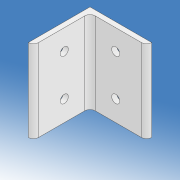
# Autodesk Inventor part: NASA-20-EBOX-EXT-CB-01
Saved by Autodesk Inventor 2020 (Build 240168000, 168)
## iProperties
Created: 2019-12-04
Part Number: NASA-20-EBOX-EXT-CB-01
Material: Generic
Document SubType Name: Modeling
Designer: mpark
Density: 1 g/cm^3
Appearance: White
Author: mpark
Autodesk Inventor part; units mm, degrees
ref_plane "YZ Plane" through (0, 0, 0) normal (1, 0, 0) x (0, 1, 0)
ref_plane "XZ Plane" through (0, 0, 0) normal (0, 1, 0) x (-1, 0, 0)
ref_plane "XY Plane" through (0, 0, 0) normal (0, 0, 1) x (1, 0, 0)
sketch "Sketch1" plane through (0, 0, 0) normal (0, 1, 0) x (-1, 0, 0)
  line L0 (-38.1, 0) -> (0, 0)
  line L1 (0, 0) -> (0, 38.1)
  line L2 (-34.925, 3.175) -> (-6.35, 3.175)
  line L3 (-3.175, 6.35) -> (-3.175, 34.925)
  line L4 (0, 38.1) -> (0, 38.1)
  line L5 (-38.1, 0) -> (-38.1, 0)
  arc A0 (0, 38.1) -> (-3.175, 34.925) centre (0, 34.925) ccw
  arc A1 (-34.925, 3.175) -> (-38.1, 0) centre (-34.925, 0) ccw
  arc A2 (-6.35, 3.175) -> (-3.175, 6.35) centre (-6.35, 6.35) ccw
  point P0 (0, 38.1)
  dimension "d0" = 38.1
  dimension "d1" = 38.1
  dimension "d2" = 3.175
  dimension "d3" = 3.175
  constraints: 12 end point, 6 point on circle, 6 tangent, 3 centre point, 3 perpendicular, 2 equal radius, 2 horizontal, 1 other
  measures "d0" distance of L0.end L1.end
  measures "d1" distance of L0.start L0.end
  measures "d2" distance between parallel lines of L0 L2
  measures "d3" radius of A0
extrude "Extrusion1" add sketch "Sketch1" along normal blind 50.8
sketch "Sketch2" plane through (38.1, 0, 0) normal (0, 0, -1) x (-1, 0, 0)
  line L0 (0, 0) -> (38.1, 0) projected
  line L1 (38.1, 0) -> (38.1, 50.8) projected
  line L2 (0, 50.8) -> (38.1, 50.8) projected
  line L3 (0, 0) -> (0, 50.8) projected
  point P0 (19.05, 38.1)
  point P1 (19.05, 12.7)
  dimension "d6" = 12.7
  dimension "d7" = 12.7
  dimension "d8" = 19.05
  constraints: 1 vertical alignment
  measures "d6" distance from line of point (19.05, 12.7) L0
  measures "d7" distance from line of L2 point (19.05, 38.1)
  measures "d8" distance from line of L1 point (19.05, 38.1)
hole "Hole1" at (19.05, 38.1, 0) at (19.05, 12.7, 0) direction (0, 0, 1) diameter 5 end through all
sketch "Sketch3" plane through (0, 0, 0) normal (-1, 0, 0) x (0, 0, 1)
  line L0 (0, 0) -> (38.1, 0) projected
  line L1 (38.1, 0) -> (38.1, 50.8) projected
  line L2 (0, 50.8) -> (38.1, 50.8) projected
  line L3 (0, 0) -> (0, 50.8) projected
  point P0 (19.05, 38.1)
  point P1 (19.05, 12.7)
  dimension "d16" = 12.7
  dimension "d17" = 12.7
  dimension "d18" = 19.05
  constraints: 1 vertical alignment
  measures "d16" distance from line of L2 point (19.05, 38.1)
  measures "d17" distance from line of L0 point (19.05, 12.7)
  measures "d18" distance from line of point (19.05, 38.1) L1
hole "Hole2" at (0, 38.1, 19.05) at (0, 12.7, 19.05) direction (1, 0, 0) diameter 5 end through all
equation "\"d7\" = d6"
equation "\"d17\" = d16"
body "Solid1"
